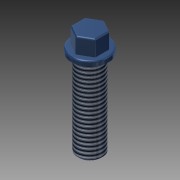
# Autodesk Inventor part: 装填斗固定螺丝
Saved by Autodesk Inventor 2015 (Build 190159000, 159)
## iProperties
Created: 2017-05-19
Part Number: 装填斗固定螺丝
Material: 常规
Document SubType Name: Modeling
Designer: Administrator
Density: 1 g/cm^3
Appearance: 薄片缎光 - 蓝色
Author: Administrator
Autodesk Inventor part; units mm, degrees
ref_plane "YZ Plane" through (0, 0, 0) normal (1, 0, 0) x (0, 1, 0)
ref_plane "XZ Plane" through (0, 0, 0) normal (0, 1, 0) x (-1, 0, 0)
ref_plane "XY Plane" through (0, 0, 0) normal (0, 0, 1) x (1, 0, 0)
sketch "草图1" plane through (0, 0, 0) normal (0, 0, 1) x (1, 0, 0)
  circle A0 centre (0, 0) radius 6
  dimension "d0" = 12
  constraints: 1 centre point, 1 coincident
  measures "d0" diameter of A0
extrude "拉伸1" add sketch "草图1" along normal blind 1.5
sketch "草图2" plane through (0, 0, 1.5) normal (0, 0, 1) x (1, 0, 0)
  line L0 (0, -4.6188) -> (-4, -2.3094)
  line L1 (-4, -2.3094) -> (-4, 2.3094)
  line L2 (-4, 2.3094) -> (0, 4.6188)
  line L3 (0, 4.6188) -> (4, 2.3094)
  line L4 (4, 2.3094) -> (4, -2.3094)
  line L5 (4, -2.3094) -> (0, -4.6188)
  line L6 (0, 0) -> (0, 2.9591)
  dimension "d3" = 8
  dimension "d4" = 2.9591
  constraints: 14 end point, 1 coincident, 1 point on line, 1 vertical, 13 other
  measures "d3" distance between parallel lines of L5 L2
  measures "d4" distance of L6.start L6.end
extrude "拉伸2" add sketch "草图2" along normal blind 5
sketch "草图3" plane through (0, 0, 0) normal (0, 0, -1) x (-1, 0, 0)
  circle A0 centre (0, 0) radius 4
  dimension "d7" = 8
  constraints: 1 centre point, 1 coincident
  measures "d7" diameter of A0
extrude "拉伸3" add sketch "草图3" along normal blind 28
thread "螺纹1" size "M8x1.25" class "6g" standard "ANSI Metric M Profile" full length
chamfer "倒角1" distance 0.5 angle 45 1 edges at (4, 0, -28)
fillet "圆角1" radius 0.5 13 edges at (-6, 0, 1.5) (4, 0, 6.5) (2, 3.4641, 6.5) (-2, 3.4641, 6.5) (-4, 0, 6.5) (-2, -3.4641, 6.5) (2, -3.4641, 6.5) (4, 2.3094, 4) (0, 4.6188, 4) (4, -2.3094, 4) (0, -4.6188, 4) (-4, -2.3094, 4) (-4, 2.3094, 4)
